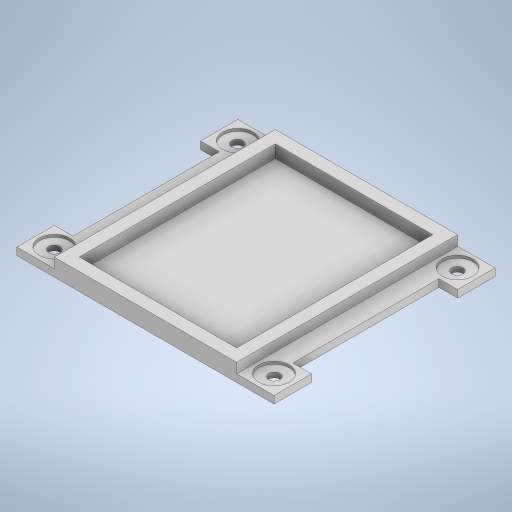
# Autodesk Inventor part: battery_pack_base
Saved by Autodesk Inventor 2023 (Build 270158000, 158)
## iProperties
Created: 2024-04-12
Part Number: battery_pack_base
Material: Genérico
Document SubType Name: Modeling
Designer: inigo
Density: 1 g/cm^3
Appearance: Valor por defecto
Author: inigo
Autodesk Inventor part; units mm, degrees
ref_plane "YZ Plane" through (0, 0, 0) normal (1, 0, 0) x (0, 1, 0)
ref_plane "XZ Plane" through (0, 0, 0) normal (0, 1, 0) x (-1, 0, 0)
ref_plane "XY Plane" through (0, 0, 0) normal (0, 0, 1) x (1, 0, 0)
sketch "Boceto1" plane through (0, 0, 0) normal (0, 1, 0) x (-1, 0, 0)
  line L0 (-31.6, 39.35) -> (-31.6, -39.25)
  line L1 (-31.6, -39.25) -> (31.5, -39.25)
  line L2 (31.5, -39.25) -> (31.5, 39.35)
  line L3 (31.5, 39.35) -> (-31.6, 39.35)
  line L4 (-31.6, 39.35) -> (31.5, -39.25) construction
  line L5 (-31.6, -39.25) -> (31.5, 39.35) construction
  line L6 (36.5, 44.35) -> (36.5, -44.25)
  line L7 (36.5, -44.25) -> (-36.6, -44.25)
  line L8 (-36.6, -44.25) -> (-36.6, 44.35)
  line L9 (-36.6, 44.35) -> (36.5, 44.35)
  point P0 (0, 0)
  point P1 (-0.05, 0.05)
  dimension "d0" = 78.6
  dimension "d1" = 63.1
  dimension "d2" = 5
  constraints: 20 end point, 4 parallel, 2 midpoint, 2 perpendicular, 3 other
  measures "d0" distance of L2.end L1.end
  measures "d1" distance of L1.end L0.end
  measures "d2" distance between parallel lines of L2 L6
extrude "Extrusión1" add sketch "Boceto1" along normal blind 2 contours L3 L2 L1 L0
sketch "Boceto2" plane through (0, 0, 0) normal (0, 1, 0) x (-1, 0, 0)
  line L0 (-31.6, 39.35) -> (-31.6, -39.25)
  line L1 (-31.6, -39.25) -> (31.5, -39.25)
  line L2 (31.5, -39.25) -> (31.5, 39.35)
  line L3 (31.5, 39.35) -> (-31.6, 39.35)
  line L4 (-31.6, 39.35) -> (31.5, -39.25) construction
  line L5 (-31.6, -39.25) -> (31.5, 39.35) construction
  line L6 (36.5, 44.35) -> (36.5, -44.25)
  line L7 (36.5, -44.25) -> (-36.6, -44.25)
  line L8 (-36.6, -44.25) -> (-36.6, 44.35)
  line L9 (-36.6, 44.35) -> (36.5, 44.35)
  point P0 (0, 0)
  point P1 (0, 0)
  point P2 (-0.05, 0.05)
  dimension "d5" = 78.6
  dimension "d6" = 63.1
  dimension "d7" = 5
  constraints: 20 end point, 4 parallel, 2 midpoint, 2 perpendicular, 3 other
  measures "d5" distance of L2.end L1.end
  measures "d6" distance of L1.end L0.end
  measures "d7" distance between parallel lines of L2 L6
extrude "Extrusión2" add sketch "Boceto2" along normal blind 7
sketch "Boceto3" plane through (0, 0, 0) normal (0, 1, 0) x (-1, 0, 0)
  circle A0 centre (44, 36.85) radius 6.1
  line L0 (36.5, 44.35) -> (-36.6, 44.35) projected
  line L1 (36.5, 44.35) -> (51.5, 44.35)
  line L2 (51.5, 44.35) -> (51.5, 29.35)
  line L3 (51.5, 29.35) -> (36.5, 29.35)
  line L4 (36.5, 29.35) -> (36.5, 44.35)
  line L5 (36.5, -44.25) -> (36.5, 44.35) projected
  line L6 (36.5, 0.05) -> (47.8738, 0.05)
  line L7 (-0.05, 44.35) -> (-0.05, 26.6285)
  circle A1 centre (44, -36.75) radius 6.1
  line L8 (36.5, -44.25) -> (51.5, -44.25)
  line L9 (51.5, -44.25) -> (51.5, -29.25)
  line L10 (51.5, -29.25) -> (36.5, -29.25)
  line L11 (36.5, -29.25) -> (36.5, -44.25)
  circle A2 centre (-44.1, 36.85) radius 6.1
  line L12 (-36.6, 44.35) -> (-51.6, 44.35)
  line L13 (-51.6, 44.35) -> (-51.6, 29.35)
  line L14 (-51.6, 29.35) -> (-36.6, 29.35)
  line L15 (-36.6, 29.35) -> (-36.6, 44.35)
  circle A3 centre (-44.1, -36.75) radius 6.1
  line L16 (-36.6, -44.25) -> (-51.6, -44.25)
  line L17 (-51.6, -44.25) -> (-51.6, -29.25)
  line L18 (-51.6, -29.25) -> (-36.6, -29.25)
  line L19 (-36.6, -29.25) -> (-36.6, -44.25)
  line L20 (44, 29.35) -> (36.5, 29.35)
  line L21 (36.5, 29.35) -> (36.5, -29.25)
  line L22 (36.5, -29.25) -> (44, -29.25)
  line L23 (44, -29.25) -> (44, 29.35)
  line L24 (-36.6, 0.05) -> (-47.9738, 0.05)
  line L25 (-36.6, 29.35) -> (-36.6, -29.25)
  line L26 (-44.1, -29.25) -> (-44.1, 29.35)
  point P0 (0, 0)
  dimension "d10" = 12.2
  dimension "d11" = 15
  dimension "d12" = 15
  constraints: 50 end point, 18 symmetric about line, 4 centre point, 4 parallel, 3 horizontal, 3 midpoint, 2 perpendicular, 1 vertical, 3 other
  measures "d10" diameter of A0
  measures "d11" distance of L2.end L3.end
  measures "d12" distance of L1.end L2.end
extrude "Extrusión3" add sketch "Boceto3" along normal blind 3 contours A0 | L15 L14 L13 L12 | L1 L2 L3 L4 | L3 L23 L6 L5 | L6 L23 L10 L5 | L25 L24 L26 L14 | L10 L9 L8 L5 | L25 L18 L26 L24 | L19 L16 L17 L18 | A1 | A2 | A3
sketch "Boceto4" plane through (0, 3, 0) normal (0, 1, 0) x (1, 0, 0)
  circle A0 centre (44, 36.85) radius 6.1
  line L0 (36.5, 44.35) -> (-36.6, 44.35)
  line L1 (36.5, 44.35) -> (51.5, 44.35)
  line L2 (51.5, 44.35) -> (51.5, 29.35)
  line L3 (51.5, 29.35) -> (36.5, 29.35)
  line L4 (36.5, 29.35) -> (36.5, 44.35)
  line L5 (36.5, -44.25) -> (36.5, 44.35)
  line L6 (36.5, 0.05) -> (47.8738, 0.05)
  line L7 (-0.05, 44.35) -> (-0.05, 26.6285)
  circle A1 centre (44, -36.75) radius 6.1
  line L8 (36.5, -44.25) -> (51.5, -44.25)
  line L9 (51.5, -44.25) -> (51.5, -29.25)
  line L10 (51.5, -29.25) -> (36.5, -29.25)
  line L11 (36.5, -29.25) -> (36.5, -44.25)
  line L12 (-51.6, 29.35) -> (-36.6, 29.35)
  circle A2 centre (-44.1, 36.85) radius 6.1
  line L13 (-36.6, 44.35) -> (-51.6, 44.35)
  line L14 (-36.6, 29.35) -> (-36.6, 44.35)
  line L15 (-51.6, 44.35) -> (-51.6, 29.35)
  line L16 (-51.6, -29.25) -> (-36.6, -29.25)
  circle A3 centre (-44.1, -36.75) radius 6.1
  line L17 (-36.6, -29.25) -> (-36.6, -44.25)
  line L18 (-51.6, -44.25) -> (-51.6, -29.25)
  line L19 (-36.6, -44.25) -> (-51.6, -44.25)
  point P0 (0, 0)
  point P1 (0, 0)
  dimension "d15" = 12.2
  dimension "d16" = 15
  dimension "d17" = 15
  constraints: 40 end point, 13 symmetric about line, 4 centre point, 2 horizontal, 2 midpoint, 2 parallel, 1 perpendicular, 1 vertical, 3 other
  measures "d15" diameter of A0
  measures "d16" distance of L2.end L4.start
  measures "d17" distance of L1.end L2.end
extrude "Extrusión4" cut sketch "Boceto4" against normal blind 1 contours A0 | A1 | A2 | A3
sketch "Boceto5" plane through (-44.1, 2, 36.75) normal (0, 1, 0) x (1, 0, 0)
  circle A0 centre (0, 0) radius 2.25
  line L0 (7.6, 66) -> (7.6, 7.4) projected
  line L1 (7.6, 36.7) -> (1.3256, 36.7)
  line L2 (44.1, -8.1109) -> (44.1, -20.0015)
  circle A1 centre (0, 73.4) radius 2.25
  circle A2 centre (88.2, 0) radius 2.25
  circle A3 centre (88.2, 73.4) radius 2.25
  point P0 (44.1, 36.75)
  dimension "d20" = 4.5
  constraints: 4 centre point, 4 end point, 3 symmetric about line, 1 horizontal, 1 midpoint, 1 vertical, 3 other
  measures "d20" diameter of A0
extrude "Extrusión5" cut sketch "Boceto5" against normal blind 2
